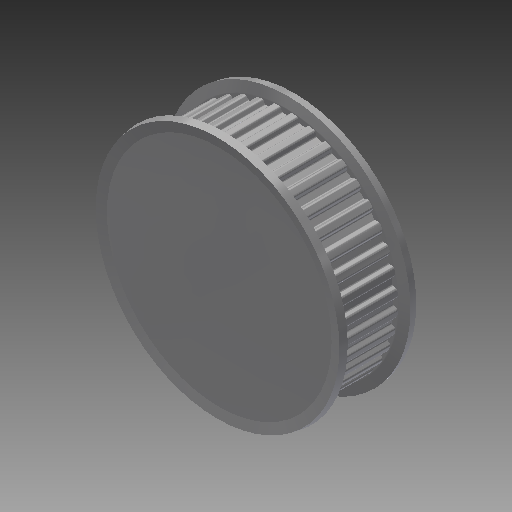
# Autodesk Inventor part: Synchronous Pulley2
Saved by Autodesk Inventor 2019.4 (Build 234330000, 330)
## iProperties
Created: 2019-12-14
Part Number: Synchronous Pulley2
Material: Steel
Document SubType Name: Modeling
Designer: admin
Density: 1 g/cm^3
Appearance: Steel
CustomPartVersion: 1
Author: admin
Autodesk Inventor part; units mm, degrees
ref_plane "YZ Plane" through (0, 0, 0) normal (1, 0, 0) x (0, 1, 0)
ref_plane "XZ Plane" through (0, 0, 0) normal (0, 1, 0) x (-1, 0, 0)
ref_plane "XY Plane" through (0, 0, 0) normal (0, 0, 1) x (1, 0, 0)
sketch "Pulley Sketch" plane through (0, 0, 0) normal (0, 0, 1) x (1, 0, 0)
  circle A0 centre (0, 0) radius 31.831 construction
  circle A1 centre (0, 0) radius 31.331
  circle A2 centre (0, 0) radius 30.081
  line L0 (-1.4669, 31.2966) -> (-0.9, 30.081)
  line L1 (-0.9, 30.081) -> (0.9, 30.081)
  line L2 (0.9, 30.081) -> (1.4669, 31.2966)
  line L3 (0, 0) -> (0, 31.331) construction
  point P0 (0, 30.081)
  dimension "d0" = 63.662
  dimension "d1" = 0.5
  dimension "d2" = 1.25
  dimension "d3" = 50
  dimension "d4" = 1.8
  constraints: 8 end point, 3 coincident, 3 point on circle, 2 centre point, 1 horizontal, 1 midpoint, 1 point on line, 1 vertical, 1 vertical alignment, 3 other
  measures "d0" diameter of A0
  measures "d1" radial gap between concentric circles of A0 A1
  measures "d3" angle of L2 L0
  measures "d4" distance of L0.end L1.end
extrude "Base Body" add sketch "Pulley Sketch" along normal mid plane 16.5 contours A2 | A1 L0 L1 L2 | L2 L1 L0 A1
extrude "Tooth" cut sketch "Pulley Sketch" along normal through all both and the other way through all contours L2 L1 L0 A1 picked at (0, 30.9118)
fillet "Tooth Fillet" radius 0.4 2 edges at (0.9, 30.081, 0) (-0.9, 30.081, 0)
fillet "Tooth Fillet" radius 0.6 4 edges at (-1.4669, 31.2966, 4.125) (-1.4669, 31.2966, -4.125) (1.4669, 31.2966, 4.125) (1.4669, 31.2966, -4.125)
pattern_circular "Teeth" count 40 over 360 about axis through (0, 0, -10) along (0, 0, 1) of "Tooth", "Tooth Fillet"
pulley flange "Left flange" diameter 62.662 height 3 thickness 2 bend angle 10 centre (0, 0, -8.25) toward (0, 0, -1)
pulley flange "Right flange" diameter 62.662 height 3 thickness 2 bend angle 10 centre (0, 0, 8.25) toward (0, 0, 1)
equation "\"d1\" = da_a"
equation "\"d2\" = da_hg"
equation "\"d3\" = 2 * da_fi"
equation "\"d4\" = da_bw"
equation "\"d5\" = da_bf"
equation "\"d7\" = da_bf"
equation "\"d9\" = da_rb"
equation "\"d10\" = da_rt"
equation "\"da_pb\" = 5"
equation "\"da_fi\" = 25deg"
equation "\"da_hg\" = 1.25"
equation "\"da_bw\" = 1.8"
equation "\"da_rb\" = 0.4"
equation "\"da_rt\" = 0.6"
equation "\"da_a\" = 0.5"
equation "\"da_bf\" = 16.5"
equation "\"da_wf\" = 2"
equation "\"da_hf\" = 3"
body "Solid1"
